Autodesk Inventor part; units mm, degrees
(part 2 of 2)
  spline S134 degree 4 poles (18.1995, -12.5936) (18.0147, -12.4624) (17.8426, -12.3149) (17.664, -12.1551) (17.6232, -11.9189) knots 1 1 1 1 1 2 2 2 2 2
  line L418 (18.0147, -12.4624) -> (17.8426, -12.3149) construction
  line L419 (17.8426, -12.3149) -> (17.664, -12.1551) construction
  line L420 (17.664, -12.1551) -> (17.6232, -11.9189) construction
  arc A71 (17.6232, -11.9189) -> (17.9434, -11.4312) centre (0, 0) ccw
  arc A72 (17.9434, -11.4312) -> (18.2501, -10.9349) centre (0, 0) ccw
  spline S135 degree 4 poles (19.1051, -11.172) (18.9081, -11.06) (18.7017, -10.9664) (18.4814, -10.8721) (18.2501, -10.9349) knots 1 1 1 1 1 2 2 2 2 2
  line L421 (19.1051, -11.172) -> (18.9081, -11.06) construction
  line L422 (18.9081, -11.06) -> (18.7017, -10.9664) construction
  line L423 (18.7017, -10.9664) -> (18.4814, -10.8721) construction
  line L424 (18.4814, -10.8721) -> (18.2501, -10.9349) construction
  line L425 (22.8279, -7.8195) -> (21.4814, -7.8186) construction
  spline S136 degree 2 poles (22.8279, -7.8195) (21.4814, -7.8186) (20.7548, -7.6847) knots 1 1 1 2 2 2
  line L426 (21.4814, -7.8186) -> (20.7548, -7.6847) construction
  spline S137 degree 2 poles (21.671, -10.6126) (20.7182, -9.6611) (20.1098, -9.242) knots 1 1 1 2 2 2
  line L427 (21.671, -10.6126) -> (20.7182, -9.6611) construction
  line L428 (20.7182, -9.6611) -> (20.1098, -9.242) construction
  line L429 (20.1098, -9.242) -> (19.9051, -9.1449) construction
  spline S138 degree 4 poles (20.1098, -9.242) (19.9051, -9.1449) (19.71, -9.0295) (19.5064, -8.9031) (19.4252, -8.6776) knots 1 1 1 1 1 2 2 2 2 2
  line L430 (19.9051, -9.1449) -> (19.71, -9.0295) construction
  line L431 (19.71, -9.0295) -> (19.5064, -8.9031) construction
  line L432 (19.5064, -8.9031) -> (19.4252, -8.6776) construction
  arc A73 (19.4252, -8.6776) -> (19.6558, -8.1417) centre (0, 0) ccw
  arc A74 (19.6558, -8.1417) -> (19.8717, -7.5997) centre (0, 0) ccw
  spline S139 degree 4 poles (20.7548, -7.6847) (20.5414, -7.6086) (20.3219, -7.5523) (20.0885, -7.4976) (19.8717, -7.5997) knots 1 1 1 1 1 2 2 2 2 2
  line L433 (20.7548, -7.6847) -> (20.5414, -7.6086) construction
  line L434 (20.5414, -7.6086) -> (20.3219, -7.5523) construction
  line L435 (20.3219, -7.5523) -> (20.0885, -7.4976) construction
  line L436 (20.0885, -7.4976) -> (19.8717, -7.5997) construction
  line L437 (23.8389, -3.7366) -> (22.5127, -3.9696) construction
  spline S140 degree 2 poles (23.8389, -3.7366) (22.5127, -3.9696) (21.774, -3.9639) knots 1 1 1 2 2 2
  line L438 (22.5127, -3.9696) -> (21.774, -3.9639) construction
  spline S141 degree 2 poles (23.1846, -6.6882) (22.0811, -5.9166) (21.4092, -5.6095) knots 1 1 1 2 2 2
  line L439 (23.1846, -6.6882) -> (22.0811, -5.9166) construction
  line L440 (22.0811, -5.9166) -> (21.4092, -5.6095) construction
  line L441 (21.4092, -5.6095) -> (21.1907, -5.5495) construction
  spline S142 degree 4 poles (21.4092, -5.6095) (21.1907, -5.5495) (20.9785, -5.4697) (20.756, -5.3806) (20.6369, -5.1726) knots 1 1 1 1 1 2 2 2 2 2
  line L442 (21.1907, -5.5495) -> (20.9785, -5.4697) construction
  line L443 (20.9785, -5.4697) -> (20.756, -5.3806) construction
  line L444 (20.756, -5.3806) -> (20.6369, -5.1726) construction
  arc A75 (20.6369, -5.1726) -> (20.771, -4.6048) centre (0, 0) ccw
  arc A76 (20.771, -4.6048) -> (20.8894, -4.0336) centre (0, 0) ccw
  spline S143 degree 4 poles (21.774, -3.9639) (21.5506, -3.926) (21.3246, -3.9087) (21.0853, -3.8954) (20.8894, -4.0336) knots 1 1 1 1 1 2 2 2 2 2
  line L445 (21.774, -3.9639) -> (21.5506, -3.926) construction
  line L446 (21.5506, -3.926) -> (21.3246, -3.9087) construction
  line L447 (21.3246, -3.9087) -> (21.0853, -3.8954) construction
  line L448 (21.0853, -3.8954) -> (20.8894, -4.0336) construction
  circle A77 centre (0, 0) radius 24.13
  point P0 (21.1615, 2.1976)
  point P1 (20.4584, 5.8389)
  point P2 (17.2276, 12.4839)
  point P3 (14.7981, 15.2858)
  point P4 (11.9189, 17.6232)
  point P5 (5.1726, 20.6369)
  point P6 (1.5105, 21.2216)
  point P7 (-5.8389, 20.4584)
  point P8 (-12.4839, 17.2276)
  point P9 (-15.2858, 14.7981)
  point P10 (-17.6232, 11.9189)
  point P11 (-19.4252, 8.6776)
  point P12 (-20.6369, 5.1726)
  point P13 (-21.2216, 1.5105)
  point P14 (-20.4584, -5.8389)
  point P15 (-17.2276, -12.4839)
  point P16 (-14.7981, -15.2858)
  point P17 (-11.9189, -17.6232)
  point P18 (-8.6776, -19.4252)
  point P19 (-5.1726, -20.6369)
  point P20 (-1.5105, -21.2216)
  point P21 (2.1976, -21.1615)
  point P22 (5.8389, -20.4584)
  point P23 (12.4839, -17.2276)
  point P24 (15.2858, -14.7981)
  point P25 (17.6232, -11.9189)
  point P26 (20.6369, -5.1726)
  point P27 (21.2216, -1.5105)
  dimension "d0" = 45.72
  dimension "d1" = 1.27
  dimension "d2" = 14.5
  dimension "d3" = 5.7237
  dimension "d4" = 5.7237
  dimension "d5" = 9.6145
  dimension "d6" = 3.8908
  dimension "d10" = 21.2725
  dimension "d13" = 75.5
  dimension "d14" = 75.5
  dimension "d15" = 21.2725
  dimension "d16" = 75.5
  dimension "d17" = 21.2725
  dimension "d18" = 75.5
  dimension "d19" = 21.2725
  dimension "d20" = 2.5
  dimension "d23" = 360
  constraints: 152 point on circle, 76 centre point, 34 end point, 13 coincident, 9 symmetric about line, 5 point on line, 3 collinear, 3 equal length, 2 concentric, 1 horizontal, 1 perpendicular, 1 tangent, 1 vertical, 1709 other
  measures "d0" diameter of A0
  measures "d2" angle of L1 L0
  measures "d3" distance of L1.end L2.end
  measures "d5" distance of L4.start L4.end
  measures "d10" distance from line of point (0, 0) L5
  measures "d13" angle of L5 L6
  measures "d14" angle of L7 L8
  measures "d15" distance from line of point (0, 0) L7
  measures "d16" angle of L10 L11
  measures "d17" distance from line of point (0, 0) L10
  measures "d18" angle of L13 L14
  measures "d19" distance from line of point (0, 0) L13
  measures "d20" angle of L0 L16
extrude "Extrusion1" add sketch "Sketch1" along normal blind 9.525 contours A5 S3 S2 A77 S140 S143 A76 A75 S142 S141 S136 S139 A74 A73 S138 S137 S132 S135 A72 A71 S134 S133 S128 S131 A70 A69 S130 S129 S124 S127 A68 A67 S126 S125 S120 S123 A66 A65 S122 S121 S116 S119 A64 A63 S118 S117 S112 S115 A62 A61 S114 S113 S108 S111 A60 A59 S110 S109 S104 S107 A58 A57 S106 S105 S100 S103 A56 A55 S102 S101 S96 S99 A54 A53 S98 S97 S92 S95 A52 A51 S94 S93 S88 S91 A50 A49 S90 S89 S84 S87 A48 A47 S86 S85 S80 S83 A46 A45 S82 S81 S76 S79 A44 A43 S78 S77 S72 S75 A42 A41 S74 S73 S68 S71 A40 A39 S70 S69 S64 S67 A38 A37 S66 S65 S60 S63 A36 A35 S62 S61 S56 S59 A34 A33 S58 S57 S52 S55 A32 A31 S54 S53 S48 S51 A30 A29 S50 S49 S44 S47 A28 A27 S46 S45 S40 S43 A26 A25 S42 S41 S36 S39 A24 A23 S38 S37 S32 S35 A22 A21 S34 S33 S28 S31 A20 A19 S30 S29 S24 S27 A18 A17 S26 S25 S20 S23 A16 A15 S22 S21 S16 S19 A14 A13 S18 S17 S12 S15 A12 A11 S14 S13 S8 S11 A10 A9 S10 S9 S4 S7 A8 A7 S6 S5 S0 S1 A4
sketch "Sketch2" plane through (0, 9.525, 0) normal (0, 1, 0) x (1, 0, 0)
  arc A0 (-24.1256, -0.4597) -> (-24.0739, -1.6447) centre (0, 0) ccw projected
  arc A1 (-21.1615, -2.1976) -> (-21.0092, -3.3543) centre (0, 0) ccw projected
  arc A2 (-23.6793, -4.6421) -> (-23.4225, -5.8001) centre (0, 0) ccw projected
  arc A3 (-20.4584, -5.8389) -> (-20.1076, -6.9515) centre (0, 0) ccw projected
  arc A4 (-22.5134, -8.6834) -> (-22.0595, -9.7793) centre (0, 0) ccw projected
  arc A5 (-19.1337, -9.3027) -> (-18.595, -10.3376) centre (0, 0) ccw projected
  arc A6 (-20.6635, -12.4609) -> (-20.0262, -13.4613) centre (0, 0) ccw projected
  arc A7 (-17.2276, -12.4839) -> (-16.5174, -13.4095) centre (0, 0) ccw projected
  arc A8 (-18.1858, -15.8598) -> (-17.3845, -16.7343) centre (0, 0) ccw projected
  arc A9 (-14.7981, -15.2858) -> (-13.9379, -16.074) centre (0, 0) ccw projected
  arc A10 (-15.1555, -18.7768) -> (-14.2145, -19.4989) centre (0, 0) ccw projected
  arc A11 (-11.9189, -17.6232) -> (-10.9349, -18.2501) centre (0, 0) ccw projected
  arc A12 (-11.6647, -21.1233) -> (-10.6126, -21.671) centre (0, 0) ccw projected
  arc A13 (-8.6776, -19.4252) -> (-7.5997, -19.8717) centre (0, 0) ccw projected
  arc A14 (-7.8195, -22.8279) -> (-6.6882, -23.1846) centre (0, 0) ccw projected
  arc A15 (-5.1726, -20.6369) -> (-4.0336, -20.8894) centre (0, 0) ccw projected
  arc A16 (-3.7366, -23.8389) -> (-2.5606, -23.9937) centre (0, 0) ccw projected
  arc A17 (-1.5105, -21.2216) -> (-0.3449, -21.2725) centre (0, 0) ccw projected
  arc A18 (0.4597, -24.1256) -> (1.6447, -24.0739) centre (0, 0) ccw projected
  arc A19 (2.1976, -21.1615) -> (3.3543, -21.0092) centre (0, 0) ccw projected
  arc A20 (4.6421, -23.6793) -> (5.8001, -23.4225) centre (0, 0) ccw projected
  arc A21 (5.8389, -20.4584) -> (6.9515, -20.1076) centre (0, 0) ccw projected
  arc A22 (8.6834, -22.5134) -> (9.7793, -22.0595) centre (0, 0) ccw projected
  arc A23 (9.3027, -19.1337) -> (10.3376, -18.595) centre (0, 0) ccw projected
  arc A24 (12.4609, -20.6635) -> (13.4613, -20.0262) centre (0, 0) ccw projected
  arc A25 (12.4839, -17.2276) -> (13.4095, -16.5174) centre (0, 0) ccw projected
  arc A26 (15.8598, -18.1858) -> (16.7343, -17.3845) centre (0, 0) ccw projected
  arc A27 (15.2858, -14.7981) -> (16.074, -13.9379) centre (0, 0) ccw projected
  arc A28 (18.7768, -15.1555) -> (19.4989, -14.2145) centre (0, 0) ccw projected
  arc A29 (17.6232, -11.9189) -> (18.2501, -10.9349) centre (0, 0) ccw projected
  arc A30 (21.1233, -11.6647) -> (21.671, -10.6126) centre (0, 0) ccw projected
  arc A31 (19.4252, -8.6776) -> (19.8717, -7.5997) centre (0, 0) ccw projected
  arc A32 (22.8279, -7.8195) -> (23.1846, -6.6882) centre (0, 0) ccw projected
  arc A33 (20.6369, -5.1726) -> (20.8894, -4.0336) centre (0, 0) ccw projected
  arc A34 (23.8389, -3.7366) -> (23.9937, -2.5606) centre (0, 0) ccw projected
  arc A35 (21.2216, -1.5105) -> (21.2725, -0.3449) centre (0, 0) ccw projected
  arc A36 (24.1256, 0.4597) -> (24.0739, 1.6447) centre (0, 0) ccw projected
  arc A37 (21.1615, 2.1976) -> (21.0092, 3.3543) centre (0, 0) ccw projected
  arc A38 (23.6793, 4.6421) -> (23.4225, 5.8001) centre (0, 0) ccw projected
  arc A39 (20.4584, 5.8389) -> (20.1076, 6.9515) centre (0, 0) ccw projected
  arc A40 (22.5134, 8.6834) -> (22.0595, 9.7793) centre (0, 0) ccw projected
  arc A41 (19.1337, 9.3027) -> (18.595, 10.3376) centre (0, 0) ccw projected
  arc A42 (20.6635, 12.4609) -> (20.0262, 13.4613) centre (0, 0) ccw projected
  arc A43 (17.2276, 12.4839) -> (16.5174, 13.4095) centre (0, 0) ccw projected
  arc A44 (18.1858, 15.8598) -> (17.3845, 16.7343) centre (0, 0) ccw projected
  arc A45 (14.7981, 15.2858) -> (13.9379, 16.074) centre (0, 0) ccw projected
  arc A46 (15.1555, 18.7768) -> (14.2145, 19.4989) centre (0, 0) ccw projected
  arc A47 (11.9189, 17.6232) -> (10.9349, 18.2501) centre (0, 0) ccw projected
  arc A48 (11.6647, 21.1233) -> (10.6126, 21.671) centre (0, 0) ccw projected
  arc A49 (8.6776, 19.4252) -> (7.5997, 19.8717) centre (0, 0) ccw projected
  arc A50 (7.8195, 22.8279) -> (6.6882, 23.1846) centre (0, 0) ccw projected
  arc A51 (5.1726, 20.6369) -> (4.0336, 20.8894) centre (0, 0) ccw projected
  arc A52 (3.7366, 23.8389) -> (2.5606, 23.9937) centre (0, 0) ccw projected
  arc A53 (1.5105, 21.2216) -> (0.3449, 21.2725) centre (0, 0) ccw projected
  arc A54 (-0.4597, 24.1256) -> (-1.6447, 24.0739) centre (0, 0) ccw projected
  arc A55 (-2.1976, 21.1615) -> (-3.3543, 21.0092) centre (0, 0) ccw projected
  arc A56 (-4.6421, 23.6793) -> (-5.8001, 23.4225) centre (0, 0) ccw projected
  arc A57 (-5.8389, 20.4584) -> (-6.9515, 20.1076) centre (0, 0) ccw projected
  arc A58 (-8.6834, 22.5134) -> (-9.7793, 22.0595) centre (0, 0) ccw projected
  arc A59 (-9.3027, 19.1337) -> (-10.3376, 18.595) centre (0, 0) ccw projected
  arc A60 (-12.4609, 20.6635) -> (-13.4613, 20.0262) centre (0, 0) ccw projected
  arc A61 (-12.4839, 17.2276) -> (-13.4095, 16.5174) centre (0, 0) ccw projected
  arc A62 (-15.8598, 18.1858) -> (-16.7343, 17.3845) centre (0, 0) ccw projected
  arc A63 (-15.2858, 14.7981) -> (-16.074, 13.9379) centre (0, 0) ccw projected
  arc A64 (-18.7768, 15.1555) -> (-19.4989, 14.2145) centre (0, 0) ccw projected
  arc A65 (-17.6232, 11.9189) -> (-18.2501, 10.9349) centre (0, 0) ccw projected
  arc A66 (-21.1233, 11.6647) -> (-21.671, 10.6126) centre (0, 0) ccw projected
  arc A67 (-19.4252, 8.6776) -> (-19.8717, 7.5997) centre (0, 0) ccw projected
  arc A68 (-22.8279, 7.8195) -> (-23.1846, 6.6882) centre (0, 0) ccw projected
  arc A69 (-20.6369, 5.1726) -> (-20.8894, 4.0336) centre (0, 0) ccw projected
  arc A70 (-23.8389, 3.7366) -> (-23.9937, 2.5606) centre (0, 0) ccw projected
  arc A71 (-21.2216, 1.5105) -> (-21.2725, 0.3449) centre (0, 0) ccw projected
  circle A72 centre (0, 0) radius 19.1008 construction
  line L0 (0, 0) -> (-17.5098, 2.3052) construction
  line L1 (0, 0) -> (-18.2308, 0) construction
  arc A73 (-18.226, 0.4165) -> (-18.2308, 0) centre (0, 0) ccw
  arc A74 (-17.732, 0.8319) -> (-18.226, 0.4165) centre (-17.7962, 0.4067) ccw
  arc A75 (-17.732, 0.8319) -> (-16.0325, 2.1107) centre (-17.5098, 2.3052) ccw
  line L2 (-18.9374, 2.4932) -> (-18.9374, 2.4932) construction
  arc A76 (-17.6096, 4.7185) -> (-17.7128, 4.3149) centre (0, 0) ccw
  arc A77 (-17.7128, 4.3149) -> (-17.3431, 3.7859) centre (-17.295, 4.2132) ccw
  arc A78 (-16.0325, 2.1107) -> (-17.3431, 3.7859) centre (-17.5098, 2.3052) ccw
  arc A79 (-17.7128, -4.3149) -> (-17.6096, -4.7185) centre (0, 0) ccw
  arc A80 (-17.3431, -3.7859) -> (-17.7128, -4.3149) centre (-17.295, -4.2132) ccw
  arc A81 (-17.3431, -3.7859) -> (-16.0325, -2.1107) centre (-17.5098, -2.3052) ccw
  arc A82 (-16.0325, -2.1107) -> (-17.732, -0.8319) centre (-17.5098, -2.3052) ccw
  arc A83 (-18.226, -0.4165) -> (-17.732, -0.8319) centre (-17.7962, -0.4067) ccw
  arc A84 (-18.2308, 0) -> (-18.226, -0.4165) centre (0, 0) ccw
  arc A85 (-15.9925, -8.7523) -> (-15.7883, -9.1154) centre (0, 0) ccw
  arc A86 (-15.7723, -8.1456) -> (-15.9925, -8.7523) centre (-15.6153, -8.5459) ccw
  arc A87 (-15.7723, -8.1456) -> (-14.9399, -6.1883) centre (-16.3165, -6.7585) ccw
  arc A88 (-14.9399, -6.1883) -> (-16.9125, -5.3929) centre (-16.3165, -6.7585) ccw
  arc A89 (-17.4972, -5.1196) -> (-16.9125, -5.3929) centre (-17.0845, -4.9988) ccw
  arc A90 (-17.6096, -4.7185) -> (-17.4972, -5.1196) centre (0, 0) ccw
  arc A91 (-13.1823, -12.5932) -> (-12.8911, -12.8911) centre (0, 0) ccw
  arc A92 (-13.1267, -11.9502) -> (-13.1823, -12.5932) centre (-12.8713, -12.2962) ccw
  arc A93 (-13.1267, -11.9502) -> (-12.8292, -9.8442) centre (-14.0113, -10.7513) ccw
  arc A94 (-12.8292, -9.8442) -> (-14.9404, -9.5864) centre (-14.0113, -10.7513) ccw
  arc A95 (-15.576, -9.4737) -> (-14.9404, -9.5864) centre (-15.2086, -9.2503) ccw
  arc A96 (-15.7883, -9.1154) -> (-15.576, -9.4737) centre (0, 0) ccw
  arc A97 (-9.4737, -15.576) -> (-9.1154, -15.7883) centre (0, 0) ccw
  arc A98 (-9.5864, -14.9404) -> (-9.4737, -15.576) centre (-9.2503, -15.2086) ccw
  arc A99 (-9.5864, -14.9404) -> (-9.8442, -12.8292) centre (-10.7513, -14.0113) ccw
  arc A100 (-9.8442, -12.8292) -> (-11.9502, -13.1267) centre (-10.7513, -14.0113) ccw
  arc A101 (-12.5932, -13.1823) -> (-11.9502, -13.1267) centre (-12.2962, -12.8713) ccw
  arc A102 (-12.8911, -12.8911) -> (-12.5932, -13.1823) centre (0, 0) ccw
  arc A103 (-5.1196, -17.4972) -> (-4.7185, -17.6096) centre (0, 0) ccw
  arc A104 (-5.3929, -16.9125) -> (-5.1196, -17.4972) centre (-4.9988, -17.0845) ccw
  arc A105 (-5.3929, -16.9125) -> (-6.1883, -14.9399) centre (-6.7585, -16.3165) ccw
  arc A106 (-6.1883, -14.9399) -> (-8.1456, -15.7723) centre (-6.7585, -16.3165) ccw
  arc A107 (-8.7523, -15.9925) -> (-8.1456, -15.7723) centre (-8.5459, -15.6153) ccw
  arc A108 (-9.1154, -15.7883) -> (-8.7523, -15.9925) centre (0, 0) ccw
  arc A109 (-0.4165, -18.226) -> (0, -18.2308) centre (0, 0) ccw
  arc A110 (-0.8319, -17.732) -> (-0.4165, -18.226) centre (-0.4067, -17.7962) ccw
  arc A111 (-0.8319, -17.732) -> (-2.1107, -16.0325) centre (-2.3052, -17.5098) ccw
  arc A112 (-2.1107, -16.0325) -> (-3.7859, -17.3431) centre (-2.3052, -17.5098) ccw
  arc A113 (-4.3149, -17.7128) -> (-3.7859, -17.3431) centre (-4.2132, -17.295) ccw
  arc A114 (-4.7185, -17.6096) -> (-4.3149, -17.7128) centre (0, 0) ccw
  arc A115 (4.3149, -17.7128) -> (4.7185, -17.6096) centre (0, 0) ccw
  arc A116 (3.7859, -17.3431) -> (4.3149, -17.7128) centre (4.2132, -17.295) ccw
  arc A117 (3.7859, -17.3431) -> (2.1107, -16.0325) centre (2.3052, -17.5098) ccw
  arc A118 (2.1107, -16.0325) -> (0.8319, -17.732) centre (2.3052, -17.5098) ccw
  arc A119 (0.4165, -18.226) -> (0.8319, -17.732) centre (0.4067, -17.7962) ccw
  arc A120 (0, -18.2308) -> (0.4165, -18.226) centre (0, 0) ccw
  arc A121 (8.7523, -15.9925) -> (9.1154, -15.7883) centre (0, 0) ccw
  arc A122 (8.1456, -15.7723) -> (8.7523, -15.9925) centre (8.5459, -15.6153) ccw
  arc A123 (8.1456, -15.7723) -> (6.1883, -14.9399) centre (6.7585, -16.3165) ccw
  arc A124 (6.1883, -14.9399) -> (5.3929, -16.9125) centre (6.7585, -16.3165) ccw
  arc A125 (5.1196, -17.4972) -> (5.3929, -16.9125) centre (4.9988, -17.0845) ccw
  arc A126 (4.7185, -17.6096) -> (5.1196, -17.4972) centre (0, 0) ccw
  arc A127 (12.5932, -13.1823) -> (12.8911, -12.8911) centre (0, 0) ccw
  arc A128 (11.9502, -13.1267) -> (12.5932, -13.1823) centre (12.2962, -12.8713) ccw
  arc A129 (11.9502, -13.1267) -> (9.8442, -12.8292) centre (10.7513, -14.0113) ccw
  arc A130 (9.8442, -12.8292) -> (9.5864, -14.9404) centre (10.7513, -14.0113) ccw
  arc A131 (9.4737, -15.576) -> (9.5864, -14.9404) centre (9.2503, -15.2086) ccw
  arc A132 (9.1154, -15.7883) -> (9.4737, -15.576) centre (0, 0) ccw
  arc A133 (15.576, -9.4737) -> (15.7883, -9.1154) centre (0, 0) ccw
  arc A134 (14.9404, -9.5864) -> (15.576, -9.4737) centre (15.2086, -9.2503) ccw
  arc A135 (14.9404, -9.5864) -> (12.8292, -9.8442) centre (14.0113, -10.7513) ccw
  arc A136 (12.8292, -9.8442) -> (13.1267, -11.9502) centre (14.0113, -10.7513) ccw
  arc A137 (13.1823, -12.5932) -> (13.1267, -11.9502) centre (12.8713, -12.2962) ccw
  arc A138 (12.8911, -12.8911) -> (13.1823, -12.5932) centre (0, 0) ccw
  arc A139 (17.4972, -5.1196) -> (17.6096, -4.7185) centre (0, 0) ccw
  arc A140 (16.9125, -5.3929) -> (17.4972, -5.1196) centre (17.0845, -4.9988) ccw
  arc A141 (16.9125, -5.3929) -> (14.9399, -6.1883) centre (16.3165, -6.7585) ccw
  arc A142 (14.9399, -6.1883) -> (15.7723, -8.1456) centre (16.3165, -6.7585) ccw
  arc A143 (15.9925, -8.7523) -> (15.7723, -8.1456) centre (15.6153, -8.5459) ccw
  arc A144 (15.7883, -9.1154) -> (15.9925, -8.7523) centre (0, 0) ccw
  arc A145 (18.226, -0.4165) -> (18.2308, 0) centre (0, 0) ccw
  arc A146 (17.732, -0.8319) -> (18.226, -0.4165) centre (17.7962, -0.4067) ccw
  arc A147 (17.732, -0.8319) -> (16.0325, -2.1107) centre (17.5098, -2.3052) ccw
  arc A148 (16.0325, -2.1107) -> (17.3431, -3.7859) centre (17.5098, -2.3052) ccw
  arc A149 (17.7128, -4.3149) -> (17.3431, -3.7859) centre (17.295, -4.2132) ccw
  arc A150 (17.6096, -4.7185) -> (17.7128, -4.3149) centre (0, 0) ccw
  arc A151 (17.7128, 4.3149) -> (17.6096, 4.7185) centre (0, 0) ccw
  arc A152 (17.3431, 3.7859) -> (17.7128, 4.3149) centre (17.295, 4.2132) ccw
  arc A153 (17.3431, 3.7859) -> (16.0325, 2.1107) centre (17.5098, 2.3052) ccw
  arc A154 (16.0325, 2.1107) -> (17.732, 0.8319) centre (17.5098, 2.3052) ccw
  arc A155 (18.226, 0.4165) -> (17.732, 0.8319) centre (17.7962, 0.4067) ccw
  arc A156 (18.2308, 0) -> (18.226, 0.4165) centre (0, 0) ccw
  arc A157 (15.9925, 8.7523) -> (15.7883, 9.1154) centre (0, 0) ccw
  arc A158 (15.7723, 8.1456) -> (15.9925, 8.7523) centre (15.6153, 8.5459) ccw
  arc A159 (15.7723, 8.1456) -> (14.9399, 6.1883) centre (16.3165, 6.7585) ccw
  arc A160 (14.9399, 6.1883) -> (16.9125, 5.3929) centre (16.3165, 6.7585) ccw
  arc A161 (17.4972, 5.1196) -> (16.9125, 5.3929) centre (17.0845, 4.9988) ccw
  arc A162 (17.6096, 4.7185) -> (17.4972, 5.1196) centre (0, 0) ccw
  arc A163 (13.1823, 12.5932) -> (12.8911, 12.8911) centre (0, 0) ccw
  arc A164 (13.1267, 11.9502) -> (13.1823, 12.5932) centre (12.8713, 12.2962) ccw
  arc A165 (13.1267, 11.9502) -> (12.8292, 9.8442) centre (14.0113, 10.7513) ccw
  arc A166 (12.8292, 9.8442) -> (14.9404, 9.5864) centre (14.0113, 10.7513) ccw
  arc A167 (15.576, 9.4737) -> (14.9404, 9.5864) centre (15.2086, 9.2503) ccw
  arc A168 (15.7883, 9.1154) -> (15.576, 9.4737) centre (0, 0) ccw
  arc A169 (9.4737, 15.576) -> (9.1154, 15.7883) centre (0, 0) ccw
  arc A170 (9.5864, 14.9404) -> (9.4737, 15.576) centre (9.2503, 15.2086) ccw
  arc A171 (9.5864, 14.9404) -> (9.8442, 12.8292) centre (10.7513, 14.0113) ccw
  arc A172 (9.8442, 12.8292) -> (11.9502, 13.1267) centre (10.7513, 14.0113) ccw
  arc A173 (12.5932, 13.1823) -> (11.9502, 13.1267) centre (12.2962, 12.8713) ccw
  arc A174 (12.8911, 12.8911) -> (12.5932, 13.1823) centre (0, 0) ccw
  arc A175 (5.1196, 17.4972) -> (4.7185, 17.6096) centre (0, 0) ccw
  arc A176 (5.3929, 16.9125) -> (5.1196, 17.4972) centre (4.9988, 17.0845) ccw
  arc A177 (5.3929, 16.9125) -> (6.1883, 14.9399) centre (6.7585, 16.3165) ccw
  arc A178 (6.1883, 14.9399) -> (8.1456, 15.7723) centre (6.7585, 16.3165) ccw
  arc A179 (8.7523, 15.9925) -> (8.1456, 15.7723) centre (8.5459, 15.6153) ccw
  arc A180 (9.1154, 15.7883) -> (8.7523, 15.9925) centre (0, 0) ccw
  arc A181 (0.4165, 18.226) -> (0, 18.2308) centre (0, 0) ccw
  arc A182 (0.8319, 17.732) -> (0.4165, 18.226) centre (0.4067, 17.7962) ccw
  arc A183 (0.8319, 17.732) -> (2.1107, 16.0325) centre (2.3052, 17.5098) ccw
  arc A184 (2.1107, 16.0325) -> (3.7859, 17.3431) centre (2.3052, 17.5098) ccw
  arc A185 (4.3149, 17.7128) -> (3.7859, 17.3431) centre (4.2132, 17.295) ccw
  arc A186 (4.7185, 17.6096) -> (4.3149, 17.7128) centre (0, 0) ccw
  arc A187 (-4.3149, 17.7128) -> (-4.7185, 17.6096) centre (0, 0) ccw
  arc A188 (-3.7859, 17.3431) -> (-4.3149, 17.7128) centre (-4.2132, 17.295) ccw
  arc A189 (-3.7859, 17.3431) -> (-2.1107, 16.0325) centre (-2.3052, 17.5098) ccw
  arc A190 (-2.1107, 16.0325) -> (-0.8319, 17.732) centre (-2.3052, 17.5098) ccw
  arc A191 (-0.4165, 18.226) -> (-0.8319, 17.732) centre (-0.4067, 17.7962) ccw
  arc A192 (0, 18.2308) -> (-0.4165, 18.226) centre (0, 0) ccw
  arc A193 (-8.7523, 15.9925) -> (-9.1154, 15.7883) centre (0, 0) ccw
  arc A194 (-8.1456, 15.7723) -> (-8.7523, 15.9925) centre (-8.5459, 15.6153) ccw
  arc A195 (-8.1456, 15.7723) -> (-6.1883, 14.9399) centre (-6.7585, 16.3165) ccw
  arc A196 (-6.1883, 14.9399) -> (-5.3929, 16.9125) centre (-6.7585, 16.3165) ccw
  arc A197 (-5.1196, 17.4972) -> (-5.3929, 16.9125) centre (-4.9988, 17.0845) ccw
  arc A198 (-4.7185, 17.6096) -> (-5.1196, 17.4972) centre (0, 0) ccw
  arc A199 (-12.5932, 13.1823) -> (-12.8911, 12.8911) centre (0, 0) ccw
  arc A200 (-11.9502, 13.1267) -> (-12.5932, 13.1823) centre (-12.2962, 12.8713) ccw
  arc A201 (-11.9502, 13.1267) -> (-9.8442, 12.8292) centre (-10.7513, 14.0113) ccw
  arc A202 (-9.8442, 12.8292) -> (-9.5864, 14.9404) centre (-10.7513, 14.0113) ccw
  arc A203 (-9.4737, 15.576) -> (-9.5864, 14.9404) centre (-9.2503, 15.2086) ccw
  arc A204 (-9.1154, 15.7883) -> (-9.4737, 15.576) centre (0, 0) ccw
  arc A205 (-15.576, 9.4737) -> (-15.7883, 9.1154) centre (0, 0) ccw
  arc A206 (-14.9404, 9.5864) -> (-15.576, 9.4737) centre (-15.2086, 9.2503) ccw
  arc A207 (-14.9404, 9.5864) -> (-12.8292, 9.8442) centre (-14.0113, 10.7513) ccw
  arc A208 (-12.8292, 9.8442) -> (-13.1267, 11.9502) centre (-14.0113, 10.7513) ccw
  arc A209 (-13.1823, 12.5932) -> (-13.1267, 11.9502) centre (-12.8713, 12.2962) ccw
  arc A210 (-12.8911, 12.8911) -> (-13.1823, 12.5932) centre (0, 0) ccw
  arc A211 (-17.4972, 5.1196) -> (-17.6096, 4.7185) centre (0, 0) ccw
  arc A212 (-16.9125, 5.3929) -> (-17.4972, 5.1196) centre (-17.0845, 4.9988) ccw
  arc A213 (-16.9125, 5.3929) -> (-14.9399, 6.1883) centre (-16.3165, 6.7585) ccw
  arc A214 (-14.9399, 6.1883) -> (-15.7723, 8.1456) centre (-16.3165, 6.7585) ccw
  arc A215 (-15.9925, 8.7523) -> (-15.7723, 8.1456) centre (-15.6153, 8.5459) ccw
  arc A216 (-15.7883, 9.1154) -> (-15.9925, 8.7523) centre (0, 0) ccw
  point P0 (-22.1315, 0.1227)
  point P1 (-22.0366, -2.0511)
  point P2 (-21.8166, -3.7222)
  point P3 (-21.3456, -5.8466)
  point P4 (-20.8388, -7.4541)
  point P5 (-20.0061, -9.4644)
  point P6 (-19.2278, -10.9595)
  point P7 (-18.0587, -12.7946)
  point P8 (-17.0326, -14.1319)
  point P9 (-15.5626, -15.7361)
  point P10 (-14.3199, -16.8748)
  point P11 (-12.5936, -18.1995)
  point P12 (-11.172, -19.1051)
  point P13 (-9.242, -20.1098)
  point P14 (-7.6847, -20.7548)
  point P15 (-5.6095, -21.4092)
  point P16 (-3.9639, -21.774)
  point P17 (-1.8066, -22.058)
  point P18 (-0.1227, -22.1315)
  point P19 (2.0511, -22.0366)
  point P20 (3.7222, -21.8166)
  point P21 (5.8466, -21.3456)
  point P22 (7.4541, -20.8388)
  point P23 (9.4644, -20.0061)
  point P24 (10.9595, -19.2278)
  point P25 (12.7946, -18.0587)
  point P26 (14.1319, -17.0326)
  point P27 (15.7361, -15.5626)
  point P28 (16.8748, -14.3199)
  point P29 (18.1995, -12.5936)
  point P30 (19.1051, -11.172)
  point P31 (20.1098, -9.242)
  point P32 (20.7548, -7.6847)
  point P33 (21.4092, -5.6095)
  point P34 (21.774, -3.9639)
  point P35 (22.058, -1.8066)
  point P36 (22.1315, -0.1227)
  point P37 (22.0366, 2.0511)
  point P38 (21.8166, 3.7222)
  point P39 (21.3456, 5.8466)
  point P40 (20.8388, 7.4541)
  point P41 (20.0061, 9.4644)
  point P42 (19.2278, 10.9595)
  point P43 (18.0587, 12.7946)
  point P44 (17.0326, 14.1319)
  point P45 (15.5626, 15.7361)
  point P46 (14.3199, 16.8748)
  point P47 (12.5936, 18.1995)
  point P48 (11.172, 19.1051)
  point P49 (9.242, 20.1098)
  point P50 (7.6847, 20.7548)
  point P51 (5.6095, 21.4092)
  point P52 (3.9639, 21.774)
  point P53 (1.8066, 22.058)
  point P54 (0.1227, 22.1315)
  point P55 (-2.0511, 22.0366)
  point P56 (-3.7222, 21.8166)
  point P57 (-5.8466, 21.3456)
  point P58 (-7.4541, 20.8388)
  point P59 (-9.4644, 20.0061)
  point P60 (-10.9595, 19.2278)
  point P61 (-12.7946, 18.0587)
  point P62 (-14.1319, 17.0326)
  point P63 (-15.7361, 15.5626)
  point P64 (-16.8748, 14.3199)
  point P65 (-18.1995, 12.5936)
  point P66 (-19.1051, 11.172)
  point P67 (-20.1098, 9.242)
  point P68 (-20.7548, 7.6847)
  point P69 (-21.4092, 5.6095)
  point P70 (-21.774, 3.9639)
  point P71 (-22.058, 1.8066)
  point P72 (-18.2308, 0)
  point P73 (-17.6096, -4.7185)
  point P74 (-15.7883, -9.1154)
  point P75 (-12.8911, -12.8911)
  point P76 (-9.1154, -15.7883)
  point P77 (-4.7185, -17.6096)
  point P78 (0, -18.2308)
  point P79 (4.7185, -17.6096)
  point P80 (9.1154, -15.7883)
  point P81 (12.8911, -12.8911)
  point P82 (15.7883, -9.1154)
  point P83 (17.6096, -4.7185)
  point P84 (18.2308, 0)
  point P85 (17.6096, 4.7185)
  point P86 (15.7883, 9.1154)
  point P87 (12.8911, 12.8911)
  point P88 (9.1154, 15.7883)
  point P89 (4.7185, 17.6096)
  point P90 (0, 18.2308)
  point P91 (-4.7185, 17.6096)
  point P92 (-9.1154, 15.7883)
  point P93 (-12.8911, 12.8911)
  point P94 (-15.7883, 9.1154)
  dimension "d27" = 38.2016
  dimension "d28" = 0.43
  dimension "d29" = 1.49
  dimension "d30" = 0.87
  dimension "d31" = 7.5
  dimension "d33" = 2.9299
  dimension "d36" = 360
  constraints: 290 point on circle, 145 centre point, 6 end point, 4 symmetric about line, 3 coincident, 3 tangent, 2 point on line, 1 concentric, 1 horizontal, 556 other
  measures "d27" diameter of A72
  measures "d28" radius of A74
  measures "d29" radius of A75
  measures "d30" radial gap between concentric circles of A73 A72
  measures "d31" angle of L1 L0
  measures "d33" distance from line of A75.end L2
extrude "Extrusion2" add sketch "Sketch2" along normal blind 10
sketch "Sketch3" plane through (0, 19.525, 0) normal (0, 1, 0) x (1, 0, 0)
  circle A0 centre (0, 0) radius 21.59
  dimension "d40" = 43.18
  constraints: 1 centre point, 1 coincident
  measures "d40" diameter of A0
extrude "Extrusion3" add sketch "Sketch3" along normal blind 0.635
sketch "Sketch4" plane through (0, 0, 0) normal (0, -1, 0) x (1, 0, 0)
  line L0 (6.35, -3.6662) -> (0, -7.3323)
  line L1 (0, -7.3323) -> (-6.35, -3.6662)
  line L2 (-6.35, -3.6662) -> (-6.35, 3.6662)
  line L3 (-6.35, 3.6662) -> (0, 7.3323)
  line L4 (0, 7.3323) -> (6.35, 3.6662)
  line L5 (6.35, 3.6662) -> (6.35, -3.6662)
  point P0 (0, 0)
  point P1 (0, 0)
  dimension "d43" = 12.7
  constraints: 12 end point, 1 coincident, 1 vertical alignment, 13 other
  measures "d43" distance between parallel lines of L2 L5
extrude "Extrusion4" cut sketch "Sketch4" against normal through all
sketch "Sketch6" plane through (0, 0, 0) normal (0, -1, 0) x (1, 0, 0)
  circle A0 centre (0, 0) radius 8.89
  line L0 (6.35, 3.6662) -> (6.35, -3.6662) projected
  line L1 (6.35, -3.6662) -> (0, -7.3323)
  line L2 (0, -7.3323) -> (-6.35, -3.6662)
  line L3 (-6.35, -3.6662) -> (-6.35, 3.6662)
  line L4 (-6.35, 3.6662) -> (0, 7.3323)
  line L5 (0, 7.3323) -> (6.35, 3.6662)
  line L6 (6.35, 3.6662) -> (6.35, -3.6662)
  point P0 (6.35, 0)
  dimension "d46" = 17.78
  constraints: 12 end point, 2 coincident, 2 midpoint, 1 centre point, 13 other
  measures "d46" diameter of A0
extrude "Extrusion5" add sketch "Sketch6" along normal blind 2.794
equation "\"d4\" = d3"
equation "\"d6\" = d5 - d3"
body "Solid1"
